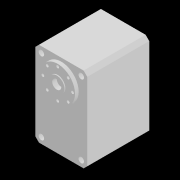
# Autodesk Inventor part: UpperArmServoDynamixelXM430-W350-T
Saved by Autodesk Inventor 2020 (Build 240168000, 168)
## iProperties
Created: 2020-03-29
Part Number: UpperArmServoDynamixelXM430-W350-T
Material: Generic
Document SubType Name: Modeling
Designer: valer
Density: 1 g/cm^3
Appearance: Default
Author: valer
Autodesk Inventor part; units mm, degrees
ref_plane "YZ Plane" through (0, 0, 0) normal (1, 0, 0) x (0, 1, 0)
ref_plane "XZ Plane" through (0, 0, 0) normal (0, 1, 0) x (-1, 0, 0)
ref_plane "XY Plane" through (0, 0, 0) normal (0, 0, 1) x (1, 0, 0)
sketch "Sketch1" plane through (0, 0, 0) normal (0, 0, 1) x (1, 0, 0)
  line L0 (-19, 24.7) -> (9.5, 24.7)
  line L1 (9.5, 24.7) -> (9.5, -21.8)
  line L2 (9.5, -21.8) -> (-19, -21.8)
  line L3 (-19, -21.8) -> (-19, 24.7)
  line L4 (-19, 21.4) -> (9.5, 21.4) construction
  line L5 (-4.75, 24.7) -> (-4.75, -21.8) construction
  circle A0 centre (-4.75, 13.27) radius 9.525
  circle A1 centre (-15.7, 21.4) radius 1.5
  line L6 (9.5, 1.45) -> (-19, 1.45) construction
  circle A2 centre (6.2, 21.4) radius 1.5
  circle A3 centre (-15.7, -18.5) radius 1.5
  circle A4 centre (6.2, -18.5) radius 1.5
  circle A5 centre (-4.75, 13.27) radius 2.5
  circle A6 centre (-4.75, 13.27) radius 4.2333
  line L7 (-4.75, 13.27) -> (-4.75, 22.795) construction
  circle A7 centre (-4.75, 21.4) radius 0.75
  circle A8 centre (-10.4988, 19.0188) radius 0.75
  circle A9 centre (-12.88, 13.27) radius 0.75
  circle A10 centre (-10.4988, 7.5212) radius 0.75
  circle A11 centre (-4.75, 5.14) radius 0.75
  circle A12 centre (0.9988, 7.5212) radius 0.75
  circle A13 centre (3.38, 13.27) radius 0.75
  circle A14 centre (0.9988, 19.0188) radius 0.75
  point P0 (0, 0)
  dimension "d2" = 19.05
  dimension "d0" = 28.5
  dimension "d1" = 46.5
  dimension "d3" = 11.43
  dimension "d4" = 3.3
  dimension "d5" = 3.3
  dimension "d6" = 3
  dimension "d7" = 5
  dimension "d8" = 8.4667
  dimension "d11" = 360
  dimension "d13" = 1.5
  constraints: 16 end point, 14 centre point, 6 point on line, 5 midpoint, 3 symmetric about line, 2 coincident, 2 horizontal, 2 parallel, 2 perpendicular, 1 vertical, 1 vertical alignment, 22 other
  measures "d0" distance of L0.start L0.end
  measures "d1" distance of L0.end L1.end
  measures "d3" distance from line of L0 point (-4.75, 13.27)
  measures "d4" distance from line of L0 A1.centre
  measures "d5" distance from line of L3 A1.centre
  measures "d6" diameter of A1
  measures "d7" diameter of A5
  measures "d8" diameter of A6
  measures "d13" diameter of A7
extrude "Extrusion1" add sketch "Sketch1" against normal blind 34 contours L0 L1 L2 L3 | A0 | A5 | A6 | A7 | A8 | A9 | A10 | A11 | A12 | A13 | A14
chamfer "Chamfer1" distance 2 angle 45 4 edges at (9.5, 24.7, -17) (-19, 24.7, -17) (9.5, -21.8, -17) (-19, -21.8, -17)
extrude "Extrusion2" add sketch "Sketch1" along normal blind 2 contours A0 | A6
extrude "Extrusion3" add sketch "Sketch1" along normal blind 2.5 contours A6
body "Solid1"
